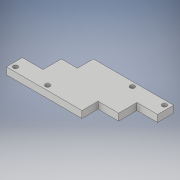
# Autodesk Inventor part: game-switch-holder
Saved by Autodesk Inventor 2017 (Build 210142000, 142)
## iProperties
Created: 2017-02-22
Part Number: game-switch-holder
Material: Generic
Document SubType Name: Modeling
Designer: John
Density: 1 g/cm^3
Appearance: Default
Author: John
Autodesk Inventor part; units mm, degrees
ref_plane "YZ Plane" through (0, 0, 0) normal (1, 0, 0) x (0, 1, 0)
ref_plane "XZ Plane" through (0, 0, 0) normal (0, 1, 0) x (-1, 0, 0)
ref_plane "XY Plane" through (0, 0, 0) normal (0, 0, 1) x (1, 0, 0)
sketch "Sketch1" plane through (0, 0, 0) normal (0, 1, 0) x (-1, 0, 0)
  line L0 (0, -7) -> (-9, -7)
  line L1 (-18, -7) -> (-18, 0)
  line L2 (-18, 0) -> (-9, 0)
  line L3 (0, 0) -> (0, -7)
  line L4 (-9, -7) -> (-9, -2) construction
  line L5 (-9, -2) -> (-9, 0) construction
  circle A0 centre (-16, -2) radius 1
  line L6 (-16, -2) -> (-9, -2) construction
  line L7 (-9, 0) -> (0, 0)
  line L8 (-9, -7) -> (-18, -7)
  circle A1 centre (-2, -2) radius 1
  circle A2 centre (-35, -20) radius 1
  line L9 (-33, -15) -> (-51, -15)
  line L10 (-51, -15) -> (-51, -22)
  line L11 (-51, -22) -> (-33, -22)
  line L12 (-33, -22) -> (-33, -15)
  line L13 (-35, -20) -> (-35, -22) construction
  line L14 (-42, -15) -> (-42, -22) construction
  circle A3 centre (-49, -20) radius 1
  line L15 (-42, -15) -> (-9, -15)
  line L16 (-9, -15) -> (-9, -7)
  line L17 (-9, -7) -> (-42, -7)
  line L18 (-42, -7) -> (-42, -15)
  line L19 (-33, -15) -> (-16, -15)
  line L20 (-16, -15) -> (-16, -22)
  line L21 (-16, -22) -> (-33, -22)
  line L22 (-33, -22) -> (-33, -15)
  line L23 (-33, -7) -> (-18, -7)
  line L24 (-18, -7) -> (-18, 0)
  line L25 (-18, 0) -> (-33, 0)
  line L26 (-33, 0) -> (-33, -7)
  point P0 (0, 0)
  dimension "d0" = 18
  dimension "d1" = 7
  dimension "d2" = 2
  dimension "d4" = 7
  dimension "d11" = 0
  dimension "d12" = 2
  dimension "d17" = 0
  dimension "d18" = 2
  dimension "d19" = 19
  dimension "d20" = 18
  dimension "d21" = 7
  dimension "d22" = 2
  dimension "d23" = 7
  dimension "d24" = 18
  dimension "d27" = 16
  dimension "d28" = 22
  constraints: 54 end point, 13 parallel, 8 perpendicular, 7 horizontal, 4 centre point, 3 point on line, 3 symmetric about line, 2 collinear, 2 midpoint, 1 coincident, 2 other
  measures "d0" distance of L1.end L3.start
  measures "d1" distance of L1.start L1.end
  measures "d2" diameter of A0
  measures "d4" distance of L6.start L4.end
  measures "d11" distance from line of point (0, 0) L2
  measures "d12" distance of L4.end L2.end
  measures "d17" distance from line of point (0, 0) L3
  measures "d18" diameter of A2
  measures "d19" horizontal distance of L13.start L6.start
  measures "d20" distance of L11.end L10.end
  measures "d21" distance of L10.end L9.end
  measures "d22" distance of L13.start L13.end
  measures "d23" distance from line of L13.start L14
  measures "d24" vertical distance of A0.centre L13.start
  measures "d27" distance between parallel lines of L20 L3
  measures "d28" distance between parallel lines of L21 L7
extrude "Extrusion2" add sketch "Sketch1" along normal blind 3
body "Solid2"
